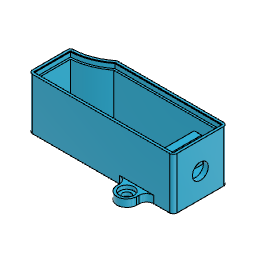
connecteur_moteur_KOSMOS3-0 (Autodesk Fusion 360 design; units mm, degrees)
Autodesk Fusion 360 part; units mm, degrees
note: some values were not read from the file. Set by a fixed rule: which sketch regions a step uses.
sketch "Esquisse1" plane through (0, 0, 0) normal (0, 0, 1) x (1, 0, 0)
  line L0 (0, 0) -> (59, 0)
  line L1 (59, 0) -> (59, 22)
  line L2 (59, 22) -> (0, 22)
  line L3 (0, 22) -> (0, 0)
  line L4 (0, 0) -> (0, 17) construction
  line L5 (0, 17) -> (0, 39) construction
  arc A0 (0, 17) -> (13.9642, 22) centre (0, 39) ccw
  dimension "d1" = 22
  dimension "d2" = 59
  dimension "d3" = 17
  dimension "d4" = 22
  constraint horizontal L0
  constraint vertical L1
  constraint horizontal L2
  constraint vertical L3
  constraint coincident L0.start L3.end
  constraint perpendicular L0 L4
  constraint perpendicular L2 L5
  constraint coincident L5.end A0.centre
  constraint coincident L2 A0.end
  measures "d1" distance of L0.start L2.end
  measures "d2" distance of L0.start L0.end
  measures "d3" distance of L0.start L4.end
  measures "d4" distance of L4.end L5.end
extrude "Extrusion1" add sketch "Esquisse1" along normal blind 2 contours L0 L1 L2 L3 A0
sketch "Esquisse2" plane through (0, 0, 2) normal (0, 0, 1) x (-1, 0, 0)
  line L0 (0, 0) -> (-59, 0)
  line L1 (-59, 0) -> (-59, -22)
  line L2 (-59, -22) -> (-13.9642, -22)
  arc A0 (0, -17) -> (-13.9642, -22) centre (0, -39) ccw
  line L3 (0, -17) -> (0, 0)
  arc A1 (-2, -15.0835) -> (-14.6629, -20) centre (0, -39) ccw
  line L4 (-57, -20) -> (-14.6629, -20)
  line L5 (-57, -2) -> (-57, -20)
  line L6 (-2, -2) -> (-57, -2)
  line L7 (-2, -15.0835) -> (-2, -2)
  dimension "d7" = -2
extrude "Extrusion2" add sketch "Esquisse2" along normal blind 19
sketch "Esquisse3" plane through (0, 0, 0) normal (-1, 0, 0) x (0, -1, 0)
  line L0 (-17, 0) -> (0, 0)
  line L1 (0, 0) -> (0, 21)
  line L2 (0, 21) -> (-17, 21)
  line L3 (-17, 21) -> (-17, 0)
  line L4 (-17, 7) -> (0, 7) construction
  circle A0 centre (-8.5, 7) radius 1.85 construction
  circle A1 centre (-8.4986, 5.15) radius 1.25
  circle A2 centre (-6.8986, 7.9263) radius 1.25
  circle A3 centre (-10.1029, 7.9237) radius 1.25
  dimension "d11" = 7
  dimension "d12" = 3.7
  dimension "d13" = 2.5
  dimension "d15" = 360
  constraint coincident L3 L4.start
  constraint coincident L1 L4.end
  constraint perpendicular L1 L4
  constraint midpoint L4 A0.centre
  constraint coincident A0 A1.centre
  measures "d11" distance of L0 L4
  measures "d12" diameter of A0
  measures "d13" diameter of A1
extrude "Extrusion3" cut sketch "Esquisse3" against normal blind 2 contours A1 | A2 | A3
sketch "Esquisse5" plane through (59, 0, 0) normal (1, 0, 0) x (0, 1, 0)
  line L0 (0, 0) -> (22, 0)
  line L1 (22, 0) -> (22, 21)
  line L2 (22, 21) -> (0, 21)
  line L3 (0, 21) -> (0, 0)
  circle A0 centre (11, 10) radius 3.25
  circle A1 centre (11, 10) radius 2
  dimension "d24" = 6.5
  dimension "d28" = 11
  dimension "d29" = 10
  dimension "d36" = 4
  constraint concentric A0 A1
  measures "d24" diameter of A0
  measures "d28" distance of L3 A0.centre
  measures "d29" distance of L0 A0.centre
  measures "d36" diameter of A1
sketch "Esquisse6" plane through (0, 0, 2) normal (0, 0, 1) x (-1, 0, 0)
  line L0 (-2, -2) -> (-57, -2)
  line L1 (-57, -2) -> (-57, -20)
  line L2 (-57, -20) -> (-14.6629, -20)
  arc A0 (-2, -15.0835) -> (-14.6629, -20) centre (0, -39) ccw
  line L3 (-2, -15.0835) -> (-2, -2)
  line L4 (-57, -20) -> (-47, -20)
  line L5 (-47, -20) -> (-47, -2)
  line L6 (-47, -2) -> (-57, -2)
  line L7 (-57, -2) -> (-57, -20)
  dimension "d25" = 10
  constraint horizontal L4
  constraint vertical L5
  constraint horizontal L6
  constraint vertical L7
  constraint coincident L1.end L2.start
  constraint coincident L0 L5.end
  measures "d25" distance of L1.end L4.end
extrude "Extrusion5" add sketch "Esquisse6" along normal blind 12 contours L0 L1 L2 L4 L5 L6 L7
extrude "Extrusion6" cut sketch "Esquisse5" against normal blind 19 contours A0 | A1
sketch "Esquisse7" plane through (0, 0, 14) normal (0, 0, 1) x (-1, 0, 0)
  line L0 (-57, -2) -> (-57, -20)
  line L1 (-57, -20) -> (-47, -20)
  line L2 (-47, -20) -> (-47, -2)
  line L3 (-57, -20) -> (-57, -2)
  line L4 (-57, -20) -> (-51, -20)
  line L5 (-51, -20) -> (-51, -2)
  line L6 (-51, -2) -> (-57, -2)
  line L7 (-57, -2) -> (-57, -20)
  line L8 (-47, -2) -> (-57, -2)
  dimension "d35" = 6
  constraint vertical L3
  constraint coincident L0.start L3.end
  constraint horizontal L4
  constraint vertical L5
  constraint horizontal L6
  constraint vertical L7
  constraint coincident L0.end L4
  constraint coincident L5.end L8
  measures "d35" distance of L0.end L4.end
extrude "Extrusion7" cut sketch "Esquisse7" against normal blind 10 contours L0 L1 L3 L4 L5 L6 L7 L8
extrude "Extrusion8" cut sketch "Esquisse5" against normal blind 13 contours A1
sketch "Esquisse8" plane through (51, 0, 0) normal (1, 0, 0) x (0, 1, 0)
  line L0 (20, 14) -> (2, 14)
  line L1 (2, 14) -> (2, 4)
  line L2 (2, 4) -> (20, 4)
  line L3 (20, 4) -> (20, 14)
  circle A0 centre (11, 10) radius 3.25
sketch "Esquisse9" plane through (0, 0, 0) normal (0, 0, -1) x (1, 0, 0)
  line L0 (59, 0) -> (0, 0)
  line L1 (0, 0) -> (0, -17)
  arc A0 (13.9642, -22) -> (0, -17) centre (0, -39) ccw
  line L2 (13.9642, -22) -> (59, -22)
  line L3 (59, -22) -> (59, 0)
  line L4 (40, 0) -> (48, 0)
  line L5 (48, 0) -> (48, 8)
  line L6 (48, 8) -> (40, 8)
  line L7 (40, 8) -> (40, 0)
  line L8 (44, 0) -> (44, 8) construction
  line L9 (59, -11) -> (19, -11) construction
  line L10 (48, -22) -> (48, -30)
  line L11 (48, -30) -> (40, -30)
  line L12 (40, -30) -> (40, -22)
  line L13 (40, -22) -> (48, -22)
  circle A1 centre (44, 4) radius 1.7
  circle A2 centre (44, -26) radius 1.7
  dimension "d39" = 8
  dimension "d40" = 8
  dimension "d41" = 15
  dimension "d44" = 3.4
  constraint horizontal L4
  constraint vertical L5
  constraint horizontal L6
  constraint vertical L7
  constraint coincident L0 L4.start
  constraint midpoint L4 L8.start
  constraint midpoint L6 L8.end
  constraint midpoint L3 L9.start
  constraint perpendicular L1 L9
  constraint symmetric L4.start L9 L12.end
  constraint symmetric L4.end L9 L10.start
  constraint symmetric L5.end L9 L10.end
  constraint symmetric L6.end L9 L11.end
  constraint midpoint L8 A1.centre
  constraint symmetric L9 A1 A2
  measures "d39" distance of L4.start L4.end
  measures "d40" distance of L4.start L6.end
  measures "d41" distance of L3 L8
  measures "d44" diameter of A1
extrude "Extrusion9" add sketch "Esquisse9" against normal blind 3 contours L0 L4 L5 L6 L7 | L2 L10 L11 L12 L13
fillet "Congé1" radius 4 4 edges at (48, -8, 1.5) (40, -8, 1.5) (48, 30, 1.5) (40, 30, 1.5)
fillet "Congé2" radius 3 4 edges at (48, 0, 1.5) (48, 22, 1.5) (40, 22, 1.5) (40, 0, 1.5)
sketch "Esquisse10" plane through (0, 0, 21) normal (0, 0, 1) x (-1, 0, 0)
  line L0 (-2, -2) -> (-2, -15.0835)
  arc A0 (-2, -15.0835) -> (-14.6629, -20) centre (0, -39) ccw
  line L1 (-14.6629, -20) -> (-57, -20)
  line L2 (-57, -20) -> (-57, -2)
  line L3 (-57, -2) -> (-2, -2)
  line L4 (0, -17) -> (0, 0)
  line L5 (0, 0) -> (-59, 0)
  line L6 (-59, 0) -> (-59, -22)
  line L7 (-59, -22) -> (-13.9642, -22)
  arc A1 (0, -17) -> (-13.9642, -22) centre (0, -39) ccw
  line L8 (-57.8, -1.2) -> (-1.2, -1.2)
  line L9 (-1.2, -1.2) -> (-1.2, -15.8311)
  arc A2 (-1.2, -15.8311) -> (-14.3875, -20.8) centre (0, -39) ccw
  line L10 (-14.3875, -20.8) -> (-57.8, -20.8)
  line L11 (-57.8, -20.8) -> (-57.8, -1.2)
  dimension "d49" = -0.8
extrude "Extrusion10" cut sketch "Esquisse10" against normal blind 2 contours L8 L9 A2 L10 L11
chamfer "Chanfrein1" distance 0.2 angle 45 5 edges at (8.1802, 17.29, 21) (36.0937, 20.8, 21) (57.8, 11, 21) (29.5, 1.2, 21) (1.2, 8.5155, 21)
fillet "Congé3" radius 1.5 3 edges at (0, 0, 10.5) (59, 0, 10.5) (59, 22, 10.5)
fillet "Congé4" radius 1 2 edges at (0, 17, 10.5) (13.9642, 22, 10.5)
chamfer "Chanfrein2" distance 0.5 angle 45 2 edges at (51, 11, 14) (47, 11, 14)
hole "Perçage1" at (44, -4, 3) direction (0, 0, -1) diameter 6 depth 1.5 tip angle 180
hole "Perçage2" at (44, 26, 3) direction (0, 0, -1) diameter 6 depth 1.5 tip angle 180
